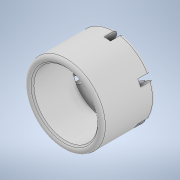
# Autodesk Inventor part: Github Test Part
Saved by Autodesk Inventor 2020 (Build 240168000, 168)
## iProperties
Created: 2021-02-03
Part Number: Github Test Part
Material: Generic
Document SubType Name: Modeling
Designer: sidsa
Density: 1 g/cm^3
Appearance: Default
Author: sidsa
Autodesk Inventor part; units mm, degrees
ref_plane "YZ Plane" through (0, 0, 0) normal (1, 0, 0) x (0, 1, 0)
ref_plane "XZ Plane" through (0, 0, 0) normal (0, 1, 0) x (-1, 0, 0)
ref_plane "XY Plane" through (0, 0, 0) normal (0, 0, 1) x (1, 0, 0)
sketch "Sketch1" plane through (0, 0, 0) normal (0, 0, 1) x (1, 0, 0)
  circle A0 centre (0, 0) radius 15.5308
  constraints: 1 centre point, 1 coincident
extrude "Extrusion1" add sketch "Sketch1" along normal blind 25.4
sketch "Sketch2" plane through (0, 0, 0) normal (0, 0, -1) x (-1, 0, 0)
  point P0 (0, 0)
sketch "Sketch3" plane through (0, 0, 25.4) normal (0, 0, 1) x (1, 0, 0)
  circle A0 centre (0, 0) radius 12.7
  dimension "d2" = 25.4
  constraints: 1 centre point, 1 coincident
  measures "d2" diameter of A0
extrude "Extrusion2" cut sketch "Sketch3" against normal blind 25.4
sketch "Sketch4" plane through (0, 0, 25.4) normal (0, 0, 1) x (1, 0, 0)
  circle A0 centre (0, 0) radius 13.97
  dimension "d5" = 27.94
  constraints: 1 centre point, 1 coincident
  measures "d5" diameter of A0
extrude "Extrusion3" cut sketch "Sketch4" against normal blind 5.08
fillet "Fillet1" radius 3.175 1 edges at (-13.97, 0, 20.32)
fillet "Fillet2" radius 3.175 1 edges at (-13.97, 0, 25.4)
fillet "Fillet3" radius 1.27 1 edges at (-15.5308, 0, 25.4)
fillet "Fillet4" radius 1.27 1 edges at (-12.7, 0, 0)
sketch "Sketch5" plane through (0, 0, 0) normal (0, 0, -1) x (-1, 0, 0)
  circle A0 centre (0, 0) radius 12.7
  constraints: 1 centre point, 1 coincident
extrude "Extrusion4" add sketch "Sketch5" against normal blind 5.08
fillet "Fillet5" radius 1.27 1 edges at (12.7, 0, 0)
sketch "Sketch6" plane through (0, 0, 0) normal (0, 0, -1) x (-1, 0, 0)
  circle A0 centre (0, 0) radius 3.175
  dimension "d15" = 6.35
  constraints: 1 centre point, 1 coincident
  measures "d15" diameter of A0
extrude "Extrusion5" cut sketch "Sketch6" against normal blind 5.08
fillet "Fillet6" radius 1.27 1 edges at (-15.5308, 0, 0)
sketch "Sketch7" plane through (0, 0, 5.08) normal (0, 0, 1) x (1, 0, 0)
  line L0 (0, 0) -> (2.54, 0)
  line L1 (2.54, 0) -> (2.54, 18.3256)
  line L2 (2.54, 18.3256) -> (0, 18.3256)
  line L3 (0, 18.3256) -> (0, 0)
  line L4 (-15.8705, 9.1628) -> (0, 0)
  line L5 (-14.6005, 11.3625) -> (-15.8705, 9.1628)
  line L6 (1.27, 2.1997) -> (-14.6005, 11.3625)
  line L7 (0, 0) -> (1.27, 2.1997)
  line L8 (-15.8705, -9.1628) -> (0, 0)
  line L9 (-17.1405, -6.9631) -> (-15.8705, -9.1628)
  line L10 (-1.27, 2.1997) -> (-17.1405, -6.9631)
  line L11 (0, 0) -> (-1.27, 2.1997)
  line L12 (0, -18.3256) -> (0, 0)
  line L13 (-2.54, -18.3256) -> (0, -18.3256)
  line L14 (-2.54, 0) -> (-2.54, -18.3256)
  line L15 (0, 0) -> (-2.54, 0)
  line L16 (15.8705, -9.1628) -> (0, 0)
  line L17 (14.6005, -11.3625) -> (15.8705, -9.1628)
  line L18 (-1.27, -2.1997) -> (14.6005, -11.3625)
  line L19 (0, 0) -> (-1.27, -2.1997)
  line L20 (15.8705, 9.1628) -> (0, 0)
  line L21 (17.1405, 6.9631) -> (15.8705, 9.1628)
  line L22 (1.27, -2.1997) -> (17.1405, 6.9631)
  line L23 (0, 0) -> (1.27, -2.1997)
  point P0 (0, 2.9329)
  point P1 (-2.54, 1.4665)
  point P2 (-2.54, -1.4665)
  point P3 (0, -2.9329)
  point P4 (2.54, -1.4665)
  point P5 (2.54, 1.4665)
  dimension "d19" = 2.54
  dimension "d22" = 360
  constraints: 48 end point, 2 coincident, 2 parallel, 1 horizontal, 1 perpendicular, 47 other
  measures "d19" distance of L2.end L1.end
extrude "Extrusion6" cut sketch "Sketch7" against normal blind 25.4
sketch "Sketch8" plane through (0, 0, 0) normal (0, 0, -1) x (-1, 0, 0)
  circle A0 centre (0, 0) radius 6.35
  dimension "d26" = 12.7
  constraints: 1 centre point, 1 coincident
  measures "d26" diameter of A0
extrude "Extrusion7" cut sketch "Sketch8" against normal blind 25.4
chamfer "Chamfer1" distance 3.175 angle 45 6 edges at (1.9845, -6.0319, 0) (-4.2316, -4.7346, 0) (-6.2161, 1.2974, 0) (-1.9845, 6.0319, 0) (4.2316, 4.7346, 0) (6.2161, -1.2974, 0)
body "Solid1"
